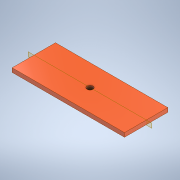
# Autodesk Inventor part: triangleBase
Saved by Autodesk Inventor 2021.1 (Build 251245010, 245A)
## iProperties
Created: 2020-11-09
Part Number: triangleBase
Material: PC/ABS Plastic
Document SubType Name: Modeling
Designer: robst
Density: 0.357273 g/cm^3
Appearance: Smooth - Light Orange
Author: robst
Autodesk Inventor part; units mm, degrees
ref_plane "YZ Plane" through (0, 0, 0) normal (1, 0, 0) x (0, 1, 0)
ref_plane "XZ Plane" through (0, 0, 0) normal (0, 1, 0) x (-1, 0, 0)
sketch "Sketch1" plane through (0, 0, 0) normal (0, 1, 0) x (-1, 0, 0)
  line L0 (88.9, 34.29) -> (-88.9, 34.29)
  line L1 (-88.9, 34.29) -> (-88.9, -34.29)
  line L2 (-88.9, -34.29) -> (88.9, -34.29)
  line L3 (88.9, -34.29) -> (88.9, 34.29)
  line L4 (88.9, 34.29) -> (-88.9, -34.29) construction
  line L5 (-88.9, 34.29) -> (88.9, -34.29) construction
  point P0 (0, 0)
  dimension "d0" = 177.8
  dimension "d1" = 68.58
  constraints: 12 end point, 2 midpoint, 2 parallel, 1 horizontal, 1 perpendicular
  measures "d0" distance of L1.end L2.end
  measures "d1" distance of L2.end L0.start
extrude "Extrusion1" add sketch "Sketch1" against normal blind 6.35
sketch "Sketch2" plane through (0, 0, 0) normal (0, 1, 0) x (1, 0, 0)
  circle A0 centre (0, 0) radius 4.7625
  dimension "d4" = 9.525
  constraints: 1 centre point, 1 coincident
  measures "d4" diameter of A0
extrude "Extrusion2" cut sketch "Sketch2" against normal through all
equation "\"d0\" = length"
equation "\"d1\" = width"
equation "\"d2\" = thickness"
equation "\"d4\" = holeDiameter"
equation "\"thickness\" = 6.35"
equation "\"length\" = 177.8"
equation "\"width\" = 68.58"
equation "\"holeDiameter\" = 9.525"
body "Solid1"
